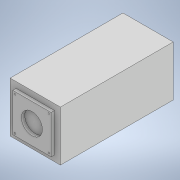
# Autodesk Inventor part: toppmt
Saved by Autodesk Inventor 2022.2 (Build 262287030, 287C)
## iProperties
Created: 2022-02-04
Part Number: toppmt
Material: Generic
Document SubType Name: Modeling
Designer: Tapendra
Density: 1 g/cm^3
Appearance: Default
Author: Tapendra
Autodesk Inventor part; units mm, degrees
ref_plane "YZ Plane" through (0, 0, 0) normal (1, 0, 0) x (0, 1, 0)
ref_plane "XZ Plane" through (0, 0, 0) normal (0, 1, 0) x (-1, 0, 0)
ref_plane "XY Plane" through (0, 0, 0) normal (0, 0, 1) x (1, 0, 0)
sketch "Sketch1" plane through (0, 0, 0) normal (0, 0, 1) x (1, 0, 0)
  line L0 (-11.25, 11.25) -> (11.25, 11.25)
  line L1 (11.25, 11.25) -> (11.25, -11.25)
  line L2 (11.25, -11.25) -> (-11.25, -11.25)
  line L3 (-11.25, -11.25) -> (-11.25, 11.25)
  line L4 (-11.25, 11.25) -> (11.25, -11.25) construction
  line L5 (11.25, 11.25) -> (-11.25, -11.25) construction
  point P0 (0, 0)
  dimension "d0" = 22.5
  dimension "d1" = 22.5
  constraints: 12 end point, 2 midpoint, 2 parallel, 1 horizontal, 1 perpendicular
  measures "d0" distance of L0.start L0.end
  measures "d1" distance of L0.end L1.end
extrude "Extrusion1" add sketch "Sketch1" along normal mid plane 50.5
sketch "Sketch3" plane through (0, 0, 25.25) normal (0, 0, 1) x (1, 0, 0)
  line L0 (-8.6, 8.6) -> (8.6, 8.6)
  line L1 (8.6, 8.6) -> (8.6, -8.6)
  line L2 (8.6, -8.6) -> (-8.6, -8.6)
  line L3 (-8.6, -8.6) -> (-8.6, 8.6)
  line L4 (-8.6, 8.6) -> (8.6, -8.6) construction
  line L5 (8.6, 8.6) -> (-8.6, -8.6) construction
  point P0 (0, 0)
  dimension "d13" = 17.2
  dimension "d14" = 17.2
  constraints: 12 end point, 2 midpoint, 2 parallel, 1 horizontal, 1 perpendicular
  measures "d13" distance of L0.start L0.end
  measures "d14" distance of L0.end L1.end
extrude "Extrusion2" add sketch "Sketch3" along normal blind 1.5
sketch "Sketch4" plane through (0, 0, 26.75) normal (0, 0, 1) x (1, 0, 0)
  circle A0 centre (-7.6, 7.6) radius 0.35 projected
  circle A1 centre (7.6, 7.6) radius 0.35 projected
  circle A2 centre (7.6, -7.6) radius 0.35 projected
  circle A3 centre (-7.6, -7.6) radius 0.35 projected
  point P0 (0, 0)
  constraints: 4 coincident
hole "Hole2" at (-7.6, 7.6, 26.75) at (7.6, 7.6, 26.75) at (7.6, -7.6, 26.75) at (-7.6, -7.6, 26.75) direction (0, 0, -1) diameter 0.7 depth 1 tip angle 118
sketch "Sketch5" plane through (0, 0, 26.75) normal (0, 0, 1) x (1, 0, 0)
  circle A0 centre (0, 0) radius 4.7128
  constraints: 1 centre point, 1 coincident
extrude "Extrusion3" cut sketch "Sketch5" against normal blind 1.5
equation "\"d14\" = d13"
body "Solid1"
